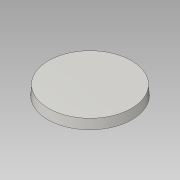
# Autodesk Inventor part: Knob (tampa)
Saved by Autodesk Inventor 2016 (Build 200138000, 138)
## iProperties
Created: 2018-09-14
Part Number: Knob (tampa)
Material: Generic
Document SubType Name: Modeling
Designer: Pedro Mendonça
Density: 1 g/cm^3
Appearance: White
Author: Pedro Mendonça
Autodesk Inventor part; units mm, degrees
ref_plane "YZ Plane" through (0, 0, 0) normal (1, 0, 0) x (0, 1, 0)
ref_plane "XZ Plane" through (0, 0, 0) normal (0, 1, 0) x (-1, 0, 0)
sketch "Sketch1" plane through (0, 0, 0) normal (0, 0, 1) x (1, 0, 0)
  circle A0 centre (0, 0) radius 8.832
  dimension "d0" = 17.664
  constraints: 1 centre point, 1 coincident
  measures "d0" diameter of A0
ref_plane "Work Plane1" through (0, 0, 2) normal (0, 0, 1) x (1, 0, 0)
sketch "Sketch2" plane through (0, 0, 2) normal (0, 0, 1) x (1, 0, 0)
  circle A0 centre (0, 0) radius 8.7
  dimension "d2" = 17.4
  constraints: 1 centre point, 1 coincident
  measures "d2" diameter of A0
loft "Loft1" add profiles "Sketch1", "Sketch2"
body "Solid1"
